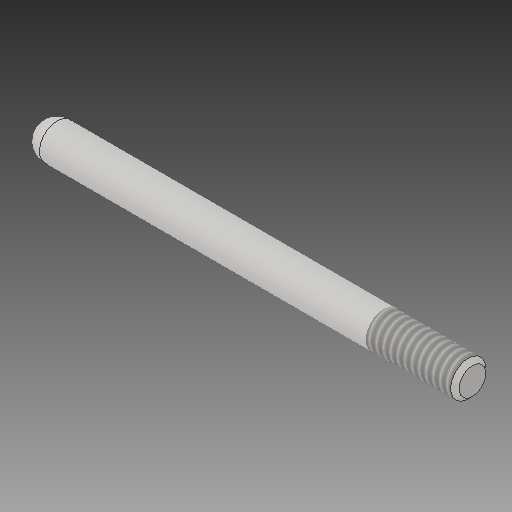
# Autodesk Inventor part: lever arm
Saved by Autodesk Inventor 2017.3 (Build 213256000, 256)
## iProperties
Created: 2017-04-20
Part Number: lever arm
Material: Generic
Document SubType Name: Modeling
Designer: 196918
Density: 1 g/cm^3
Appearance: Default
Author: 196918
Autodesk Inventor part; units mm, degrees
ref_plane "YZ Plane" through (0, 0, 0) normal (1, 0, 0) x (0, 1, 0)
ref_plane "XZ Plane" through (0, 0, 0) normal (0, 1, 0) x (-1, 0, 0)
ref_plane "XY Plane" through (0, 0, 0) normal (0, 0, 1) x (1, 0, 0)
sketch "Sketch1" plane through (0, 0, 0) normal (1, 0, 0) x (0, 1, 0)
  circle A0 centre (0, 0) radius 3.175
  dimension "d0" = 6.35
  constraints: 1 centre point, 1 coincident
  measures "d0" diameter of A0
extrude "Extrusion1" add sketch "Sketch1" along normal blind 77.7875
fillet "Fillet1" radius 3.175 1 edges at (0, -3.175, 0)
chamfer "Chamfer1" distance 0.762 angle 45 1 edges at (77.7875, -3.175, 0) measured on face at (77.7875, -0.5202, -0.7796)
thread "Thread1" size "1/4-20 UNC" class "2A" standard "ANSI Unified Screw Threads" length 15.24
body "Solid1"
